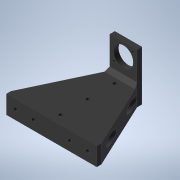
# Autodesk Inventor part: SliderLagerHalter
Saved by Autodesk Inventor 2021 (Build 250183000, 183)
## iProperties
Created: 2024-02-17
Part Number: SliderLagerHalter
Material: Generic
Document SubType Name: Modeling
Designer: Lukas
Density: 1 g/cm^3
Appearance: Default
Author: Lukas
Autodesk Inventor part; units mm, degrees
ref_plane "YZ Plane" through (0, 0, 0) normal (1, 0, 0) x (0, 1, 0)
ref_plane "XZ Plane" through (0, 0, 0) normal (0, 1, 0) x (-1, 0, 0)
ref_plane "XY Plane" through (0, 0, 0) normal (0, 0, 1) x (1, 0, 0)
sketch "Sketch1" plane through (0, 0, 0) normal (0, 1, 0) x (-1, 0, 0)
  line L0 (15, -37) -> (15, -42.5)
  line L1 (15, -42.5) -> (-15, -42.5)
  line L2 (-15, -42.5) -> (-15, -37)
  line L3 (-15, -37) -> (-50, 37.5)
  line L4 (-50, 37.5) -> (-50, 42.5)
  line L5 (-50, 42.5) -> (50, 42.5)
  line L6 (50, 42.5) -> (50, 37.5)
  line L7 (50, 37.5) -> (15, -37)
  point P0 (0, 0)
  point P1 (0, 42.5)
  point P2 (0, -42.5)
  dimension "d0" = 5
  dimension "d1" = 100
  dimension "d2" = 5.5
  dimension "d3" = 85
  dimension "d4" = 42.5
  dimension "d5" = 30
  constraints: 16 end point, 4 perpendicular, 2 equal length, 2 midpoint, 2 vertical alignment, 1 parallel, 1 vertical
  measures "d0" distance of L5.end L6.end
  measures "d1" distance of L4.end L5.end
  measures "d2" distance of L0.start L0.end
  measures "d3" distance between parallel lines of L1 L5
  measures "d4" distance from line of point (0, 0) L1
  measures "d5" distance of L0.end L1.end
extrude "Extrusion1" add sketch "Sketch1" along normal blind 20
sketch "Sketch2" plane through (15, 0, -42.5) normal (0, 0, -1) x (-1, 0, 0)
  line L0 (0, 20) -> (30, 20) projected
  line L1 (0, 20) -> (30, 20)
  line L2 (30, 20) -> (30, 55)
  line L3 (30, 55) -> (0, 55)
  line L4 (0, 55) -> (0, 20)
  line L5 (65, 0) -> (-35, 0) projected
  line L6 (-35, 0) -> (-35, 20) projected
  line L7 (65, 20) -> (-35, 20) projected
  line L8 (65, 0) -> (65, 20) projected
  circle A0 centre (-25, 10) radius 5
  circle A1 centre (-5, 10) radius 5
  circle A2 centre (35, 10) radius 5
  circle A3 centre (55, 10) radius 5
  circle A4 centre (-25, 10) radius 2.15
  circle A5 centre (-5, 10) radius 2.15
  circle A6 centre (35, 10) radius 2.15
  circle A7 centre (55, 10) radius 2.15
  point P0 (15, 0)
  point P1 (-35, 10)
  dimension "d8" = 10
  dimension "d9" = 10
  dimension "d10" = 20
  dimension "d11" = 20
  dimension "d12" = 10
  dimension "d13" = 4.3
  dimension "d22" = 35
  constraints: 8 centre point, 8 end point, 6 equal radius, 4 coincident, 4 horizontal alignment, 2 parallel, 1 horizontal, 1 midpoint, 1 perpendicular
  measures "d8" distance from line of L6 A0.centre
  measures "d9" distance from line of L8 A3.centre
  measures "d10" distance of A0.centre A1.centre
  measures "d11" distance of A3.centre A2.centre
  measures "d12" diameter of A0
  measures "d13" diameter of A4
  measures "d22" distance of L0.end L2.end
extrude "Extrusion2" cut sketch "Sketch2" against normal blind 82 contours A0 | A1 | A2 | A3 | A4 | A5 | A6 | A7
extrude "Extrusion3" cut sketch "Sketch2" against normal through all contours A4 | A5 | A6 | A7
extrude "Extrusion4" add sketch "Sketch2" against normal blind 5.5 contours L4 L3 L2 L0
sketch "Sketch3" plane through (15, 0, -37) normal (0, 0, 1) x (1, 0, 0)
  circle A0 centre (-15, 41) radius 11
  line L0 (0, 20) -> (-30, 20) projected
  circle A1 centre (-4.7652, 50.5525) radius 1.4
  circle A2 centre (-25.2348, 31.4475) radius 1.4
  line L1 (0, 0) -> (0, 55) projected
  line L2 (0, 55) -> (-30, 27)
  line L3 (-30, 55) -> (-30, 20) projected
  point P0 (-15, 0)
  point P1 (-15, 20)
  dimension "d20" = 21
  dimension "d21" = 22
  dimension "d27" = 14
  dimension "d28" = 2.8
  dimension "d29" = 14
  constraints: 3 centre point, 3 point on line, 2 end point, 2 midpoint, 1 equal radius, 1 vertical alignment
  measures "d20" distance from line of L0 A0.centre
  measures "d21" diameter of A0
  measures "d27" distance of A1.centre A0.centre
  measures "d28" diameter of A1
  measures "d29" distance of A0.centre A2.centre
extrude "Extrusion5" cut sketch "Sketch3" against normal through all contours A0 L2 | L2 A0 | L2 A1 | A1 L2 | L2 A2 | A2 L2
chamfer "Chamfer1" distance 4 angle 45 1 edges at (0, 20, -37)
sketch "Sketch4" plane through (0, 20, 0) normal (0, 1, 0) x (1, 0, 0)
  circle A0 centre (0, -32.5) radius 2.1
  circle A1 centre (0, -2.5) radius 2.1
  circle A2 centre (0, 27.5) radius 2.1
  line L0 (-50, -42.5) -> (50, -42.5) projected
  point P0 (0, 0)
  point P1 (0, -42.5)
  dimension "d33" = 4.2
  dimension "d34" = 10
  dimension "d35" = 30
  dimension "d36" = 30
  constraints: 3 centre point, 3 vertical alignment, 2 equal radius, 1 midpoint
  measures "d33" diameter of A0
  measures "d34" distance from line of L0 A0.centre
  measures "d35" distance of A1.centre A0.centre
  measures "d36" distance of A1.centre A2.centre
extrude "Extrusion6" cut sketch "Sketch4" against normal blind 10
equation "\"d4\" = 0.5 * d3"
equation "\"d9\" = d8"
equation "\"d11\" = d10"
equation "\"d29\" = d27"
body "Solid1"
